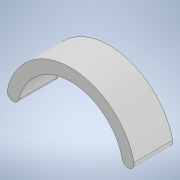
# Autodesk Inventor part: HoseClampShaftCollar
Saved by Autodesk Inventor 2020 (Build 240168000, 168)
## iProperties
Created: 2020-01-29
Part Number: HoseClampShaftCollar
Material: Generic
Document SubType Name: Modeling
Designer: srini
Density: 1 g/cm^3
Appearance: Default
Author: srini
Autodesk Inventor part; units mm, degrees
ref_plane "YZ Plane" through (0, 0, 0) normal (1, 0, 0) x (0, 1, 0)
ref_plane "XZ Plane" through (0, 0, 0) normal (0, 1, 0) x (-1, 0, 0)
ref_plane "XY Plane" through (0, 0, 0) normal (0, 0, 1) x (1, 0, 0)
sketch "Sketch1" plane through (0, 0, 0) normal (0, 0, 1) x (1, 0, 0)
  arc A0 (28.3106, 6.35) -> (-28.3106, 6.35) centre (0, 0) ccw construction
  arc A1 (31.1988, 6.9978) -> (-31.1988, 6.9978) centre (0, 0) ccw
  arc A2 (25.4224, 5.7022) -> (-25.4224, 5.7022) centre (0, 0) ccw
  arc A3 (25.4224, 5.7022) -> (31.1988, 6.9978) centre (28.3106, 6.35) ccw
  arc A4 (-31.1988, 6.9978) -> (-25.4224, 5.7022) centre (-28.3106, 6.35) ccw
  dimension "d0" = 2.96
  dimension "d1" = 26.054
  dimension "d2" = 6.35
  constraints: 10 point on circle, 5 centre point, 4 tangent, 1 coincident, 1 horizontal alignment
  measures "d0" radius of A4
  measures "d1" radius of A2
  measures "d2" vertical distance of point (0, 0) A0.end
extrude "Extrusion1" add sketch "Sketch1" along normal blind 19.05
body "Solid1"
